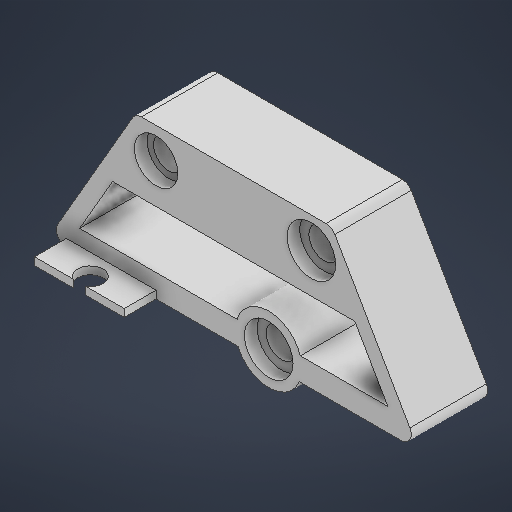
# Autodesk Inventor part: EngineMount - Big hole
Saved by Autodesk Inventor 2026.1 (Build 301233020, 233B)
## iProperties
Created: 2025-10-14
Part Number: EngineMount - Big hole
Material: Generic
Document SubType Name: Modeling
Designer: yo
Density: 1 g/cm^3
Appearance: Default
Author: yo
Autodesk Inventor part; units mm, degrees
ref_plane "YZ Plane" through (0, 0, 0) normal (1, 0, 0) x (0, 1, 0)
ref_plane "XZ Plane" through (0, 0, 0) normal (0, 1, 0) x (-1, 0, 0)
ref_plane "XY Plane" through (0, 0, 0) normal (0, 0, 1) x (1, 0, 0)
sketch "Sketch1" plane through (0, 0, 0) normal (0, 0, 1) x (1, 0, 0)
  line L0 (-65.7184, 0) -> (65.7184, 0)
  line L1 (-36.2446, 59.05) -> (36.2446, 59.05)
  circle A0 centre (-30.5, 47) radius 8.55
  line L2 (0, 59.05) -> (0, 0) construction
  circle A1 centre (-30.5, 47) radius 6
  circle A2 centre (30.5, 47) radius 6
  arc A3 (-69.1825, 6) -> (-65.7184, 0) centre (-65.7184, 4) ccw
  arc A4 (-36.2446, 59.05) -> (-39.7087, 57.05) centre (-36.2446, 55.05) ccw
  line L3 (-69.1825, 6) -> (-39.7087, 57.05)
  arc A5 (65.7184, 0) -> (69.1825, 6) centre (65.7184, 4) ccw
  arc A6 (39.7087, 57.05) -> (36.2446, 59.05) centre (36.2446, 55.05) ccw
  line L4 (69.1825, 6) -> (39.7087, 57.05)
  line L5 (-65.7184, 3) -> (-30.5, 3)
  line L6 (-30.5, 3) -> (-30.5, 0)
  line L7 (-30.5, 0) -> (-65.7184, 0)
  line L8 (-65.7184, 0) -> (-65.7184, 3)
  line L9 (-30.5, 38.45) -> (0, 38.45) construction
  line L10 (-30.5, 3) -> (0, 3) construction
  line L11 (0, 38.45) -> (0, 3) construction
  line L12 (-60.5222, 9) -> (-47.5607, 31.45)
  line L13 (-47.5607, 31.45) -> (47.5607, 31.45)
  line L14 (47.5607, 31.45) -> (60.5222, 9)
  line L15 (60.5222, 9) -> (-60.5222, 9)
  circle A7 centre (30.5, 47) radius 9.55
  circle A8 centre (13.738, 5) radius 9.55
  circle A9 centre (13.738, 5) radius 6
  line L16 (-30.5, 47) -> (13.738, 5) construction
  circle A10 centre (13.738, 5) radius 13.05
  point P0 (-65.7184, 1.5)
  point P1 (-48.1092, 0)
  point P2 (-65.7184, 0)
  point P3 (-30.5, 0)
  point P4 (-30.5, 1.5)
  point P5 (0, 20.725)
  point P6 (0, 20.725)
  point P7 (0, 20.725)
  point P8 (25.7921, 0)
  point P9 (1.6838, 0)
  point P10 (26.1598, 9)
  point P11 (1.3161, 9)
  dimension "d1" = 17.1
  dimension "d3" = 3.5
  dimension "d7" = 12
  dimension "d10" = 4
  dimension "d11" = 13
  dimension "d12" = 60
  dimension "d17" = 3
  dimension "d22" = 44
  dimension "d40" = 6
  dimension "d41" = 6
  dimension "d43" = 6
  dimension "d44" = 19.1
  dimension "d45" = 61
  dimension "d46" = 6
  dimension "d49" = 19.1
  dimension "d51" = 5
  dimension "d52" = 61
  dimension "d54" = 26.1
  constraints: 35 end point, 10 centre point, 10 coincident, 8 point on circle, 6 midpoint, 5 horizontal, 5 symmetric about line, 4 parallel, 4 tangent, 3 perpendicular, 3 vertical alignment, 2 equal radius, 2 point on line, 1 collinear, 1 horizontal alignment, 1 vertical, 5 other
  measures "d7" diameter of A1
  measures "d10" radius of A3
  measures "d11" distance from line of point (-30.5, 47) L3
  measures "d12" angle of L0 L3
  measures "d17" distance of L5.end L6.end
  measures "d22" distance from line of point (-30.5, 47) L5
  measures "d40" distance between parallel lines of L12 L3
  measures "d41" distance between parallel lines of L14 L4
  measures "d43" distance between parallel lines of L5 L15
  measures "d44" diameter of A7
  measures "d45" distance of A2.centre point (-30.5, 47)
  measures "d46" distance edge to line of A7 L13
  measures "d49" diameter of A8
  measures "d51" distance from line of A8.centre L0
  measures "d52" distance of L16.start L16.end
  measures "d54" diameter of A10
extrude "Extrusion1" add sketch "Sketch1" along normal mid plane 30 contours A3 L3 A4 L1 A6 L4 A5 L0 A10 L15 L14 L13 L12 L6 L5 L8 | A10 L15 A8 L0 | L0 A8 A10 | A10 L15 A8 | L0 A8 L15 A10
extrude "Extrusion2" add sketch "Sketch1" along normal mid plane 20 contours A8 L15 A9 L0 | L0 A9 A8 | A8 L15 A9 | L0 A9 L15 A8 | A0 | A7
extrude "Extrusion3" add sketch "Sketch1" along normal blind 27.5 contours L8 L5 L6 L0
sketch "Sketch2" plane through (-65.7184, 3, 15) normal (0, 1, 0) x (1, 0, 0)
  line L0 (0, -12.5) -> (35.2184, -12.5) projected
  arc A0 (20.1092, -12.5) -> (15.1092, -12.5) centre (17.6092, -8.1699) ccw
  line L1 (35.2184, 0) -> (131.4367, 0) construction
  line L2 (35.2184, 0) -> (35.2184, -12.5) construction
  point P0 (65.7184, 15)
  point P1 (17.6092, -12.5)
  point P2 (17.6092, -3.1699)
  dimension "d21" = 5
  dimension "d25" = 5
  constraints: 3 point on circle, 2 point on line, 1 centre point, 1 midpoint, 1 vertical alignment
  measures "d21" radius of A0
  measures "d25" distance of A0.end A0.start
extrude "Extrusion4" cut sketch "Sketch2" against normal through all
extrude "Extrusion6" add sketch "Sketch1" against normal blind 15 contours L8 L5 L6 L0
body "Solid1"
